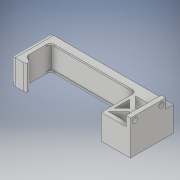
# Autodesk Inventor part: Hook Verson 2
Saved by Autodesk Inventor 2019 (Build 230136000, 136)
## iProperties
Created: 2018-11-28
Part Number: Hook Verson 2
Material: Generic
Document SubType Name: Modeling
Designer: mrhftc
Density: 1 g/cm^3
Appearance: Default
Author: mrhftc
Autodesk Inventor part; units mm, degrees
ref_plane "YZ Plane" through (0, 0, 0) normal (1, 0, 0) x (0, 1, 0)
ref_plane "XZ Plane" through (0, 0, 0) normal (0, 1, 0) x (-1, 0, 0)
ref_plane "XY Plane" through (0, 0, 0) normal (0, 0, 1) x (1, 0, 0)
sketch "Sketch1" plane through (0, 0, 0) normal (0, 1, 0) x (-1, 0, 0)
  line L0 (41.8256, 12.7) -> (-50.8, 12.7)
  line L1 (-50.8, 12.7) -> (-50.8, -16.51)
  line L2 (-50.8, -16.51) -> (41.8256, -16.51)
  line L3 (41.8256, -16.51) -> (41.8256, 12.7)
  point P0 (0, 0)
  dimension "d69" = 16.51
  dimension "d133" = 50.8
  constraints: 8 end point, 2 parallel, 1 horizontal, 1 perpendicular
  measures "d69" distance from line of L2 point (0, 0)
  measures "d133" distance from line of L1 point (0, 0)
extrude "Extrusion1" add sketch "Sketch1" along normal blind 19.05
sketch "Sketch2" plane through (0, 19.05, 0) normal (0, 1, 0) x (1, 0, 0)
  line L0 (-35.4756, -8.89) -> (29.9294, -8.89)
  line L1 (29.9294, -8.89) -> (29.9294, 7.62)
  line L2 (29.9294, 7.62) -> (-35.4756, 7.62)
  line L3 (-35.4756, 7.62) -> (-35.4756, -8.89)
  line L4 (-41.8256, 16.51) -> (-41.8256, -12.7) projected
  line L5 (-41.8256, -12.7) -> (50.8, -12.7) projected
  line L6 (50.8, -12.7) -> (50.8, 16.51) projected
  line L7 (-30.3948, -20.8465) -> (29.9294, -20.8465)
  line L8 (29.9294, -20.8465) -> (29.9294, -7.7852)
  line L9 (29.9294, -7.7852) -> (-30.3948, -7.7852)
  line L10 (-30.3948, -7.7852) -> (-30.3948, -20.8465)
  point P0 (0, 0)
  dimension "d70" = 7.62
  dimension "d92" = 3.81
  constraints: 16 end point, 4 parallel, 2 horizontal, 2 perpendicular, 1 point on line
  measures "d70" distance from line of L2 point (0, 0)
  measures "d92" distance between parallel lines of L5 L0
extrude "Extrusion2" cut sketch "Sketch2" against normal through all
sketch "Sketch23" plane through (-35.4756, 19.05, -7.62) normal (0, 0, 1) x (1, 0, 0)
  line L0 (65.405, -17.78) -> (0, -17.78)
  line L1 (0, -17.78) -> (0, -1.27)
  line L2 (0, -1.27) -> (65.405, -1.27)
  line L3 (65.405, -1.27) -> (65.405, -17.78)
  line L4 (65.405, -19.05) -> (0, -19.05) projected
  line L5 (0, 0) -> (65.405, 0) projected
  line L6 (65.405, 0) -> (65.405, -19.05) projected
  line L7 (0, 0) -> (0, -19.05) projected
  dimension "d77" = 1.27
  dimension "d78" = 1.27
  dimension "d79" = 0
  dimension "d80" = 0
  constraints: 8 end point, 2 parallel, 1 horizontal, 1 perpendicular
  measures "d77" distance between parallel lines of L4 L0
  measures "d78" distance between parallel lines of L5 L2
  measures "d79" distance between parallel lines of L6 L3
  measures "d80" distance between parallel lines of L7 L1
extrude "Extrusion8" cut sketch "Sketch23" against normal blind 3.81 contours L0 L1 L2 L3
sketch "Sketch25" plane through (0, 0, 0) normal (0, -1, 0) x (1, 0, 0)
  line L0 (-35.4756, -1.9718) -> (29.9294, -1.9718)
  line L1 (29.9294, -1.9718) -> (29.9294, -10.795)
  line L2 (29.9294, -10.795) -> (-35.4756, -10.795)
  line L3 (-35.4756, -10.795) -> (-35.4756, -1.9718)
  line L4 (-35.4756, -7.62) -> (-35.4756, 8.89) projected
  line L5 (29.9294, 12.7) -> (29.9294, -7.62) projected
  line L6 (29.9294, -7.62) -> (-35.4756, -7.62) projected
  dimension "d83" = 0
  dimension "d84" = 0
  dimension "d85" = 3.175
  constraints: 8 end point, 2 parallel, 1 horizontal, 1 perpendicular
  measures "d83" distance between parallel lines of L4 L3
  measures "d84" distance between parallel lines of L1 L5
  measures "d85" distance between parallel lines of L6 L2
extrude "Extrusion10" cut sketch "Sketch25" against normal through all
fillet "Fillet6" radius 3.175 2 edges at (-35.4756, 18.415, -10.795) (-35.4756, 0.635, -10.795)
fillet "Fillet9" radius 3.175 6 edges at (-35.4756, 9.525, 8.89) (-30.3948, 9.525, 8.89) (-30.3948, 9.525, 12.7) (-41.8256, 9.525, 12.7) (-41.8256, 19.05, -1.905) (-41.8256, 0, -1.905)
sketch "Sketch44" plane through (50.8, 0, 12.7) normal (0, 0, 1) x (1, 0, 0)
  line L0 (-20.8706, 0) -> (0, 0)
  line L1 (0, 0) -> (0, 19.05)
  line L2 (0, 19.05) -> (-20.8706, 19.05)
  line L3 (-20.8706, 19.05) -> (-20.8706, 0)
  point P0 (-50.8, 0)
  constraints: 8 end point, 2 parallel, 1 horizontal, 1 perpendicular
extrude "Extrusion19" add sketch "Sketch44" along normal blind 3.302
sketch "Sketch51" plane through (0, 19.05, 0) normal (0, 1, 0) x (1, 0, 0)
  line L0 (29.9294, 10.795) -> (50.8, 10.795)
  line L1 (50.8, 10.795) -> (50.8, -16.002)
  line L2 (50.8, -16.002) -> (29.9294, -16.002)
  line L3 (29.9294, -16.002) -> (29.9294, 10.795)
  point P0 (0, 0)
  constraints: 8 end point, 2 parallel, 1 horizontal, 1 perpendicular
extrude "Extrusion22" add sketch "Sketch51" along normal blind 7.2898
sketch "Sketch52" plane through (50.8, 0, -16.51) normal (1, 0, 0) x (0, 0, -1)
  line L0 (-26.035, 3.175) -> (0, 3.175) construction
  line L1 (-9.0678, 3.175) -> (-29.0576, 3.175)
  line L2 (-29.0576, 3.175) -> (-29.0576, 23.1648)
  line L3 (-29.0576, 23.1648) -> (-9.0678, 23.1648)
  line L4 (-9.0678, 23.1648) -> (-9.0678, 3.175)
  circle A0 centre (-29.0576, 23.1648) radius 2
  circle A1 centre (-9.0678, 23.1648) radius 2
  circle A2 centre (-9.0678, 3.175) radius 2
  circle A3 centre (-29.0576, 3.175) radius 2
  point P0 (-16.51, 0)
  constraints: 8 end point, 4 centre point, 4 coincident, 2 parallel, 1 horizontal, 1 perpendicular, 1 point on line
extrude "Extrusion23" cut sketch "Sketch52" against normal blind 25.4 contours A3 L2 L1 | L1 L2 A3 | A2 L4 L1 | L1 L4 A2 | A0 L3 L2 | L2 L3 A0 | A1 L3 L4 | L4 L3 A1
fillet "Fillet12" radius 3.175 2 edges at (29.9294, 0.635, -10.795) (29.9294, 18.415, -10.795)
sketch "Sketch53" plane through (0, 26.3398, 0) normal (0, 1, 0) x (1, 0, 0)
  line L0 (50.8, -12.827) -> (29.9294, -12.827) construction
  line L1 (29.9294, 7.62) -> (50.8, 7.62) construction
  line L2 (48.5771, 5.4422) -> (48.4734, -10.5476) construction
  line L3 (48.4734, -10.5476) -> (48.4586, -12.827) construction
  line L4 (48.5771, 5.4422) -> (48.5912, 7.62) construction
  line L5 (32.256, -12.827) -> (40.3647, -4.8829)
  line L6 (40.3647, -4.8829) -> (48.4587, -12.8126)
  line L7 (32.256, -12.827) -> (48.4587, -12.8126)
  line L8 (42.5978, -2.6035) -> (48.4875, -8.3736)
  line L9 (48.4875, -8.3736) -> (48.5622, 3.1482)
  line L10 (48.5622, 3.1482) -> (42.5978, -2.6035)
  line L11 (32.256, 7.62) -> (40.3647, -0.3241)
  line L12 (40.3647, -0.3241) -> (48.4587, 7.6056)
  line L13 (32.256, 7.62) -> (48.4587, 7.6056)
  line L14 (38.1315, -2.6035) -> (32.2419, -8.3736)
  line L15 (32.2419, -8.3736) -> (32.1672, 3.1482)
  line L16 (32.1672, 3.1482) -> (38.1315, -2.6035)
  point P0 (0, 0)
  constraints: 30 end point, 10 point on line, 1 parallel
extrude "Extrusion24" cut sketch "Sketch53" against normal through all
sketch "Sketch54" plane through (29.9294, 1.27, -11.43) normal (-1, 0, 0) x (0, 0, 1)
  line L0 (0.635, 17.78) -> (27.432, 17.78)
  line L1 (27.432, 17.78) -> (27.432, 25.0698)
  line L2 (27.432, 25.0698) -> (0.635, 25.0698)
  line L3 (0.635, 25.0698) -> (0.635, 17.78)
  point P0 (11.43, -1.27)
  constraints: 8 end point, 2 parallel, 1 horizontal, 1 perpendicular
extrude "Extrusion25" cut sketch "Sketch54" against normal blind 18.796
sketch "Sketch56" plane through (50.8, 0, -16.51) normal (1, 0, 0) x (0, 0, -1)
  line L0 (-32.512, 0) -> (-5.715, 0)
  line L1 (-5.715, 0) -> (-5.715, 26.3398)
  line L2 (-5.715, 26.3398) -> (-32.512, 26.3398)
  line L3 (-32.512, 26.3398) -> (-32.512, 0)
  line L4 (-5.715, 19.05) -> (0, 19.05)
  line L5 (0, 19.05) -> (0, 0)
  line L6 (0, 0) -> (-5.715, 0)
  line L7 (-5.715, 0) -> (-5.715, 19.05)
  point P0 (-16.51, 0)
  constraints: 16 end point, 4 parallel, 2 horizontal, 2 perpendicular
extrude "Extrusion26" add sketch "Sketch56" along normal blind 1.27
sketch "Sketch57" plane through (50.8, 23.1648, 12.5476) normal (-1, 0, 0) x (0, 0, 1)
  circle A0 centre (0, 0) radius 2 construction
  circle A1 centre (0, 0) radius 2
  point P0 (-12.5476, -23.1648)
  constraints: 1 centre point, 1 coincident, 1 concentric
extrude "Extrusion27" cut sketch "Sketch57" against normal through all
sketch "Sketch58" plane through (50.8, 23.1648, -7.4422) normal (-1, 0, 0) x (0, 0, 1)
  circle A0 centre (0, 0) radius 2 construction
  circle A1 centre (0, 0) radius 2
  point P0 (7.4422, -23.1648)
  constraints: 1 centre point, 1 coincident, 1 concentric
extrude "Extrusion28" cut sketch "Sketch58" against normal through all
body "Solid1"
